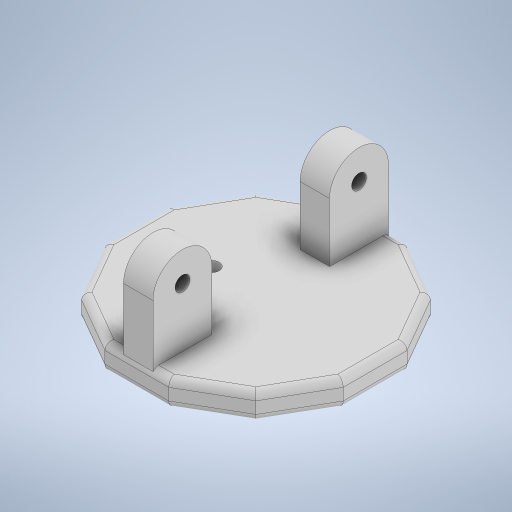
# Autodesk Inventor part: (x0.5)_POSPA_Tiny_Top
Saved by Autodesk Inventor 2024 (Build 280153000, 153)
## iProperties
Created: 2023-12-08
Part Number: (x0.5)_POSPA_Tiny_Top
Material: 일반
Document SubType Name: Modeling
Designer: jsw
Density: 1 g/cm^3
Appearance: 기본값
Author: jsw
Autodesk Inventor part; units mm, degrees
ref_plane "YZ Plane" through (0, 0, 0) normal (1, 0, 0) x (0, 1, 0)
ref_plane "XZ Plane" through (0, 0, 0) normal (0, 1, 0) x (-1, 0, 0)
ref_plane "XY Plane" through (0, 0, 0) normal (0, 0, 1) x (1, 0, 0)
sketch "스케치1" plane through (0, 0, 0) normal (0, 1, 0) x (-1, 0, 0)
  line L0 (12.4723, -12.4723) -> (4.5652, -17.0375)
  line L1 (4.5652, -17.0375) -> (-4.5652, -17.0375)
  line L2 (-4.5652, -17.0375) -> (-12.4723, -12.4723)
  line L3 (-12.4723, -12.4723) -> (-17.0375, -4.5652)
  line L4 (-17.0375, -4.5652) -> (-17.0375, 4.5652)
  line L5 (-17.0375, 4.5652) -> (-12.4723, 12.4723)
  line L6 (-12.4723, 12.4723) -> (-4.5652, 17.0375)
  line L7 (-4.5652, 17.0375) -> (4.5652, 17.0375)
  line L8 (4.5652, 17.0375) -> (12.4723, 12.4723)
  line L9 (12.4723, 12.4723) -> (17.0375, 4.5652)
  line L10 (17.0375, 4.5652) -> (17.0375, -4.5652)
  line L11 (17.0375, -4.5652) -> (12.4723, -12.4723)
  line L12 (-5.4226, 20.2375) -> (5.4226, 20.2375)
  line L13 (5.4226, 20.2375) -> (14.8149, 14.8149)
  line L14 (14.8149, 14.8149) -> (20.2375, 5.4226)
  line L15 (20.2375, 5.4226) -> (20.2375, -5.4226)
  line L16 (20.2375, -5.4226) -> (14.8149, -14.8149)
  line L17 (14.8149, -14.8149) -> (5.4226, -20.2375)
  line L18 (5.4226, -20.2375) -> (-5.4226, -20.2375)
  line L19 (-5.4226, -20.2375) -> (-14.8149, -14.8149)
  line L20 (-14.8149, -14.8149) -> (-20.2375, -5.4226)
  line L21 (-20.2375, -5.4226) -> (-20.2375, 5.4226)
  line L22 (-20.2375, 5.4226) -> (-14.8149, 14.8149)
  line L23 (-14.8149, 14.8149) -> (-5.4226, 20.2375)
  point P0 (0, 0)
  point P1 (0, 0)
  point P2 (0, 0)
  dimension "d0" = 35.277
  dimension "d1" = 3.2
  constraints: 48 end point, 2 coincident, 2 horizontal, 50 other
  measures "d0" distance of L2.end L8.end
  measures "d1" distance between parallel lines of L15 L10
extrude "돌출1" add sketch "스케치1" along normal blind 4.4 contours L0 L1 L2 L3 L4 L5 L6 L7 L8 L9 L10 L11 | L12 L13 L14 L15 L16 L17 L18 L19 L20 L21 L22 L23
sketch "스케치2" plane through (0, 4.4, 0) normal (0, 1, 0) x (1, 0, 0)
  line L0 (2.5, 10) -> (2.5, 20)
  line L1 (2.5, 20) -> (-2.5, 20)
  line L2 (-2.5, 20) -> (-2.5, 10)
  line L3 (-2.5, 10) -> (2.5, 10)
  line L4 (2.5, 10) -> (-2.5, 20) construction
  line L5 (2.5, 20) -> (-2.5, 10) construction
  line L6 (0, 0) -> (-4.4089, 0)
  line L7 (2.5, -10) -> (2.5, -20)
  line L8 (2.5, -20) -> (-2.5, -20)
  line L9 (-2.5, -20) -> (-2.5, -10)
  line L10 (-2.5, -10) -> (2.5, -10)
  line L11 (2.5, -10) -> (-2.5, -20) construction
  line L12 (2.5, -20) -> (-2.5, -10) construction
  point P0 (0, 15)
  point P1 (0, 15)
  point P2 (0, -15)
  point P3 (0, -15)
  dimension "d4" = 5
  dimension "d5" = 10
  dimension "d6" = 10
  constraints: 26 end point, 6 symmetric about line, 5 midpoint, 2 parallel, 1 horizontal, 1 perpendicular, 1 vertical, 1 vertical alignment
  measures "d4" distance of L0.end L1.end
  measures "d5" distance of L0.start L0.end
  measures "d6" distance from line of L6.start L3
extrude "돌출2" add sketch "스케치2" along normal blind 10
sketch "스케치3" plane through (2.5, 4.4, 20) normal (1, 0, 0) x (0, 0, -1)
  line L0 (40, 10) -> (30, 10) projected
  circle A0 centre (35, 10) radius 5
  line L1 (0, 10) -> (10, 10) projected
  circle A1 centre (5, 10) radius 5
  point P0 (20, -4.4)
  constraints: 2 horizontal alignment, 2 midpoint, 4 other
extrude "돌출3" add sketch "스케치3" against normal blind 5
sketch "스케치4" plane through (2.5, 4.4, 20) normal (1, 0, 0) x (0, 0, -1)
  arc A0 (10, 10) -> (0, 10) centre (5, 10) ccw projected
  circle A1 centre (5, 10) radius 1.25
  arc A2 (40, 10) -> (30, 10) centre (35, 10) ccw projected
  circle A3 centre (35, 10) radius 1.25
  point P0 (20, -4.4)
  dimension "d11" = 2.5
  dimension "d12" = 2.5
  constraints: 2 centre point, 2 coincident
  measures "d11" diameter of A1
  measures "d12" diameter of A3
extrude "돌출4" cut sketch "스케치4" against normal blind 5
fillet "모깎기1" radius 1.2 24 edges at (10.1187, 4.4, 17.5262) (17.5262, 4.4, 10.1187) (20.2375, 4.4, 0) (17.5262, 4.4, -10.1187) (10.1187, 4.4, -17.5262) (0, 4.4, -20.2375) (-10.1187, 4.4, -17.5262) (-17.5262, 4.4, -10.1187) (-20.2375, 4.4, 0) (-17.5262, 4.4, 10.1187) (-10.1187, 4.4, 17.5262) (0, 4.4, 20.2375) (-10.1187, 0, 17.5262) (-17.5262, 0, 10.1187) (-20.2375, 0, 0) (-10.1187, 0, -17.5262) (-17.5262, 0, -10.1187) (0, 0, -20.2375) (10.1187, 0, -17.5262) (17.5262, 0, -10.1187) (20.2375, 0, 0) (17.5262, 0, 10.1187) (10.1187, 0, 17.5262) (0, 0, 20.2375)
sketch "스케치5" plane through (0, 0, 0) normal (0, -1, 0) x (1, 0, 0)
  circle A0 centre (-7.5, 0) radius 1.25
  point P0 (0, 0)
  dimension "d16" = 2.5
  dimension "d17" = 7.5
  constraints: 1 centre point, 1 horizontal alignment
  measures "d16" diameter of A0
  measures "d17" distance of A0.centre point (0, 0)
extrude "돌출5" cut sketch "스케치5" against normal blind 5
sketch "스케치6" plane through (0, 0, 0) normal (0, -1, 0) x (1, 0, 0)
  line L0 (13.6436, -13.6436) -> (4.9939, -18.6375)
  line L1 (4.9939, -18.6375) -> (-4.9939, -18.6375)
  line L2 (-4.9939, -18.6375) -> (-13.6436, -13.6436)
  line L3 (-13.6436, -13.6436) -> (-18.6375, -4.9939)
  line L4 (-18.6375, -4.9939) -> (-18.6375, 4.9939)
  line L5 (-18.6375, 4.9939) -> (-13.6436, 13.6436)
  line L6 (-13.6436, 13.6436) -> (-4.9939, 18.6375)
  line L7 (-4.9939, 18.6375) -> (4.9939, 18.6375)
  line L8 (4.9939, 18.6375) -> (13.6436, 13.6436)
  line L9 (13.6436, 13.6436) -> (18.6375, 4.9939)
  line L10 (18.6375, 4.9939) -> (18.6375, -4.9939)
  line L11 (18.6375, -4.9939) -> (13.6436, -13.6436)
  line L12 (20.2375, 5.4226) -> (14.8149, 14.8149) projected
  line L13 (4.458, 16.6375) -> (12.1795, 12.1795)
  line L14 (12.1795, 12.1795) -> (16.6375, 4.458)
  line L15 (16.6375, 4.458) -> (16.6375, -4.458)
  line L16 (16.6375, -4.458) -> (12.1795, -12.1795)
  line L17 (12.1795, -12.1795) -> (4.458, -16.6375)
  line L18 (4.458, -16.6375) -> (-4.458, -16.6375)
  line L19 (-4.458, -16.6375) -> (-12.1795, -12.1795)
  line L20 (-12.1795, -12.1795) -> (-16.6375, -4.458)
  line L21 (-16.6375, -4.458) -> (-16.6375, 4.458)
  line L22 (-16.6375, 4.458) -> (-12.1795, 12.1795)
  line L23 (-12.1795, 12.1795) -> (-4.458, 16.6375)
  line L24 (-4.458, 16.6375) -> (4.458, 16.6375)
  point P0 (0, 0)
  point P1 (0, 0)
  point P2 (0, 0)
  dimension "d20" = 1.6
  dimension "d21" = 2
  constraints: 48 end point, 2 coincident, 1 horizontal, 1 vertical, 50 other
  measures "d20" distance between parallel lines of L9 L12
  measures "d21" distance between parallel lines of L9 L14
extrude "돌출6" cut sketch "스케치6" against normal blind 1.2
sketch "스케치7" plane through (0, 0, 0) normal (0, -1, 0) x (1, 0, 0)
  line L0 (16.6375, 4.458) -> (12.1795, 12.1795) projected
  line L1 (12.1795, 12.1795) -> (4.458, 16.6375) projected
  line L2 (4.458, 16.6375) -> (-4.458, 16.6375) projected
  line L3 (-4.458, 16.6375) -> (-12.1795, 12.1795) projected
  line L4 (-12.1795, 12.1795) -> (-16.6375, 4.458) projected
  line L5 (-16.6375, 4.458) -> (-16.6375, -4.458) projected
  line L6 (-16.6375, -4.458) -> (-12.1795, -12.1795) projected
  line L7 (-12.1795, -12.1795) -> (-4.458, -16.6375) projected
  line L8 (-4.458, -16.6375) -> (4.458, -16.6375) projected
  line L9 (4.458, -16.6375) -> (12.1795, -12.1795) projected
  line L10 (12.1795, -12.1795) -> (16.6375, -4.458) projected
  line L11 (16.6375, -4.458) -> (16.6375, 4.458) projected
  circle A0 centre (-7.5, 0) radius 1.25 projected
  point P0 (0, 0)
extrude "돌출7" cut sketch "스케치7" against normal blind 0.6
